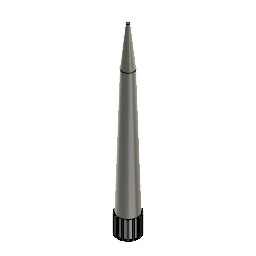
pipette_tip_remover (Autodesk Fusion 360 archive; units mm, degrees)
design "10ml_pipette_tip"
Autodesk Fusion 360 part; units mm, degrees
sketch "Sketch1" plane through (0, 0, 0) normal (0, 0, 1) x (1, 0, 0)
  circle A0 centre (0, 0) radius 8.295
  dimension "d1" = 16.59
  constraint coincident A0.centre origin
  measures "d1" diameter of A0
sketch "Sketch3" plane through (0, 0, 0) normal (0, 0, 1) x (1, 0, 0)
ref_plane "WorkPlane1" through (0, 0, 106.36) normal (0, 0, 1) x (1, 0, 0)
sketch "Sketch4" plane through (0, 0, 106.36) normal (0, 0, 1) x (1, 0, 0)
  circle A0 centre (0, 0) radius 5.07
  dimension "d4" = 10.14
  constraint coincident A0.centre origin
  measures "d4" diameter of A0
loft "Loft1" add profiles "Sketch4", "Sketch1" section 1 section 2
sketch "Sketch5" plane through (0, 0, 106.36) normal (0, 0, 1) x (-1, 0, 0)
  circle A0 centre (0, 0) radius 5.07
ref_plane "WorkPlane3" through (0, 0, 140.11) normal (0, 0, 1) x (-1, 0, 0)
sketch "Sketch6" plane through (0, 0, 140.11) normal (0, 0, 1) x (1, 0, 0)
  circle A0 centre (0, 0) radius 1.465
  dimension "d6" = 2.93
  constraint coincident A0.centre origin
  measures "d6" diameter of A0
loft "Loft2" add profiles "Sketch5", "Sketch6" section 1 section 2
sketch "Sketch7" plane through (0, 0, 0) normal (0, 0, -1) x (1, 0, 0)
  circle A0 centre (0, 0) radius 8.295
ref_plane "WorkPlane4" through (0, 0, -15.77) normal (0, 0, -1) x (1, 0, 0)
sketch "Sketch8" plane through (0, 0, -15.77) normal (0, 0, -1) x (1, 0, 0)
  circle A0 centre (0, 0) radius 9.305
  dimension "d8" = 18.61
  constraint coincident A0.centre origin
  measures "d8" diameter of A0
extrude "Extrude1" add sketch "Sketch7" along normal blind 15.77
sketch "Sketch9" plane through (0, 0, 0) normal (0, 0, 1) x (1, 0, 0)
extrude "Extrude2" add sketch "Sketch8" against normal blind 15.77
sketch "Sketch10" plane through (0, 0, 0) normal (0, 0, 1) x (-1, 0, 0)
  circle A0 centre (0, 0) radius 9.305
  circle A1 centre (0, 0) radius 8.295
  line L0 (-0.4459, 8.295) -> (0.4341, 8.295)
  line L1 (0.4341, 8.295) -> (0.4341, 10.295)
  line L2 (0.4341, 10.295) -> (-0.4459, 10.295)
  line L3 (-0.4459, 10.295) -> (-0.4459, 8.295)
  line L4 (-0.0059, 10.295) -> (-0.0059, 8.295)
  line L5 (-0.0059, 8.295) -> (-0.0059, 9.305)
  line L6 (-4.3517, 9.3407) -> (-3.5863, 7.493)
  line L7 (-3.5386, 9.6775) -> (-4.3517, 9.3407)
  line L8 (-3.5863, 7.493) -> (-2.7733, 7.8297)
  line L9 (-2.7733, 7.8297) -> (-3.5386, 9.6775)
  line L10 (-7.5949, 6.9644) -> (-6.1807, 5.5502)
  line L11 (-6.9727, 7.5866) -> (-7.5949, 6.9644)
  line L12 (-6.1807, 5.5502) -> (-5.5585, 6.1724)
  line L13 (-5.5585, 6.1724) -> (-6.9727, 7.5866)
  line L14 (-9.682, 3.5278) -> (-7.8342, 2.7624)
  line L15 (-9.3452, 4.3408) -> (-9.682, 3.5278)
  line L16 (-7.8342, 2.7624) -> (-7.4974, 3.5754)
  line L17 (-7.4974, 3.5754) -> (-9.3452, 4.3408)
  line L18 (-10.295, -0.4459) -> (-8.295, -0.4459)
  line L19 (-10.295, 0.4341) -> (-10.295, -0.4459)
  line L20 (-8.295, -0.4459) -> (-8.295, 0.4341)
  line L21 (-8.295, 0.4341) -> (-10.295, 0.4341)
  line L22 (-9.3407, -4.3517) -> (-7.493, -3.5863)
  line L23 (-9.6775, -3.5386) -> (-9.3407, -4.3517)
  line L24 (-7.493, -3.5863) -> (-7.8297, -2.7733)
  line L25 (-7.8297, -2.7733) -> (-9.6775, -3.5386)
  line L26 (-6.9644, -7.5949) -> (-5.5502, -6.1807)
  line L27 (-7.5866, -6.9727) -> (-6.9644, -7.5949)
  line L28 (-5.5502, -6.1807) -> (-6.1724, -5.5585)
  line L29 (-6.1724, -5.5585) -> (-7.5866, -6.9727)
  line L30 (-3.5278, -9.682) -> (-2.7624, -7.8342)
  line L31 (-4.3408, -9.3452) -> (-3.5278, -9.682)
  line L32 (-2.7624, -7.8342) -> (-3.5754, -7.4974)
  line L33 (-3.5754, -7.4974) -> (-4.3408, -9.3452)
  line L34 (0.4459, -10.295) -> (0.4459, -8.295)
  line L35 (-0.4341, -10.295) -> (0.4459, -10.295)
  line L36 (0.4459, -8.295) -> (-0.4341, -8.295)
  line L37 (-0.4341, -8.295) -> (-0.4341, -10.295)
  line L38 (4.3517, -9.3407) -> (3.5863, -7.493)
  line L39 (3.5386, -9.6775) -> (4.3517, -9.3407)
  line L40 (3.5863, -7.493) -> (2.7733, -7.8297)
  line L41 (2.7733, -7.8297) -> (3.5386, -9.6775)
  line L42 (7.5949, -6.9644) -> (6.1807, -5.5502)
  line L43 (6.9727, -7.5866) -> (7.5949, -6.9644)
  line L44 (6.1807, -5.5502) -> (5.5585, -6.1724)
  line L45 (5.5585, -6.1724) -> (6.9727, -7.5866)
  line L46 (9.682, -3.5278) -> (7.8342, -2.7624)
  line L47 (9.3452, -4.3408) -> (9.682, -3.5278)
  line L48 (7.8342, -2.7624) -> (7.4974, -3.5754)
  line L49 (7.4974, -3.5754) -> (9.3452, -4.3408)
  line L50 (10.295, 0.4459) -> (8.295, 0.4459)
  line L51 (10.295, -0.4341) -> (10.295, 0.4459)
  line L52 (8.295, 0.4459) -> (8.295, -0.4341)
  line L53 (8.295, -0.4341) -> (10.295, -0.4341)
  line L54 (9.3407, 4.3517) -> (7.493, 3.5863)
  line L55 (9.6775, 3.5386) -> (9.3407, 4.3517)
  line L56 (7.493, 3.5863) -> (7.8297, 2.7733)
  line L57 (7.8297, 2.7733) -> (9.6775, 3.5386)
  line L58 (6.9644, 7.5949) -> (5.5502, 6.1807)
  line L59 (7.5866, 6.9727) -> (6.9644, 7.5949)
  line L60 (5.5502, 6.1807) -> (6.1724, 5.5585)
  line L61 (6.1724, 5.5585) -> (7.5866, 6.9727)
  line L62 (3.5278, 9.682) -> (2.7624, 7.8342)
  line L63 (4.3408, 9.3452) -> (3.5278, 9.682)
  line L64 (2.7624, 7.8342) -> (3.5754, 7.4974)
  line L65 (3.5754, 7.4974) -> (4.3408, 9.3452)
  dimension "d14" = 0.88
  dimension "d15" = 2
  dimension "d17" = 360
  constraint tangent A1 L0
  constraint midpoint L2 L4.start
  constraint midpoint L0 L4.end
  constraint vertical L4
  constraint coincident L0 L4.end
  constraint coincident A1 L4.end
  constraint coincident A0 L5.end
  constraint perpendicular L0 L5
  constraint collinear L4 L5
  measures "d14" distance of L1 L3
  measures "d15" distance of L0 L2
extrude "Extrude3" cut sketch "Sketch10" against normal blind 15 contours A0 A1 L50 L52 L56 L57 | A0 A1 L46 L48 L52 L53 | A0 A1 L54 L56 L60 L61 | A0 A1 L42 L44 L48 L49 | A0 A1 L58 L60 L64 L65 | A0 A1 L38 L40 L44 L45 | A0 A1 L0 L3 L8 L9 | A0 A1 L0 L1 L62 L64 | A0 A1 L34 L36 L40 L41 | A0 A1 L30 L32 L36 L37 | A0 A1 L6 L8 L12 L13 | A0 A1 L26 L28 L32 L33 | A0 A1 L10 L12 L16 L17 | A0 A1 L22 L24 L28 L29 | A0 A1 L14 L16 L20 L21 | A0 A1 L18 L20 L24 L25
sketch "Sketch11" plane through (0, 0, -15.77) normal (0, 0, -1) x (1, 0, 0)
  circle A0 centre (0, 0) radius 9.305
  circle A1 centre (0, 0) radius 7.445
  dimension "d20" = 14.89
  constraint coincident A0.centre A1.centre
  measures "d20" diameter of A1
extrude "Extrude4" cut sketch "Sketch11" against normal blind 16 contours A1
ref_plane "WorkPlane2" through (0, 0, 106.36) normal (0, 0, 1) x (1, 0, 0)
